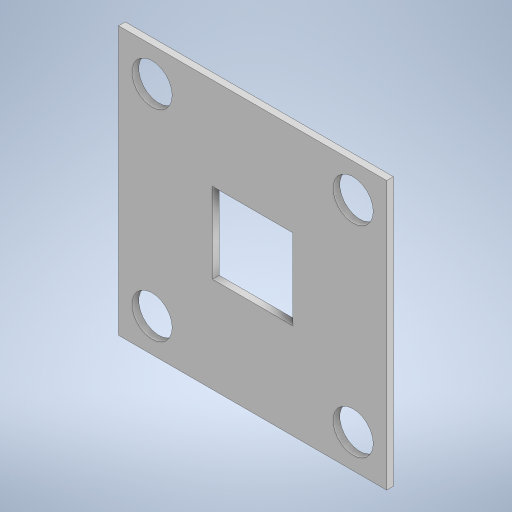
# Autodesk Inventor part: aperture12mm
Saved by Autodesk Inventor 2023 (Build 270158000, 158)
## iProperties
Created: 2022-06-22
Part Number: aperture12mm
Material: Generisch
Document SubType Name: Modeling
Designer: Tim Stechel
Density: 1 g/cm^3
Appearance: Vorgabe
Author: Tim Stechel
Autodesk Inventor part; units mm, degrees
ref_plane "YZ Plane" through (0, 0, 0) normal (1, 0, 0) x (0, 1, 0)
ref_plane "XZ Plane" through (0, 0, 0) normal (0, 1, 0) x (-1, 0, 0)
ref_plane "XY Plane" through (0, 0, 0) normal (0, 0, 1) x (1, 0, 0)
sketch "Skizze1" plane through (0, 0, 0) normal (0, 0, 1) x (1, 0, 0)
  line L0 (0, 0) -> (40, 0)
  line L1 (40, 0) -> (40, 40)
  line L2 (40, 40) -> (0, 40)
  line L3 (0, 40) -> (0, 0)
  circle A0 centre (20, 20.2527) radius 0.3489
  line L4 (0, 40) -> (5, 40)
  line L5 (0, 38.1665) -> (0, 40)
  line L6 (0, 40) -> (5, 40)
  line L7 (5, 40) -> (5, 35)
  line L8 (5, 35) -> (0, 35)
  line L9 (0, 35) -> (0, 40)
  circle A1 centre (5, 35) radius 3
  line L10 (40, 40) -> (35, 40)
  line L11 (35, 40) -> (35, 35)
  line L12 (35, 35) -> (40, 35)
  line L13 (40, 35) -> (40, 40)
  line L14 (0, 0) -> (5, 0)
  line L15 (5, 0) -> (5, 5)
  line L16 (5, 5) -> (0, 5)
  line L17 (0, 5) -> (0, 0)
  line L18 (40, 0) -> (35, 0)
  line L19 (35, 0) -> (35, 5)
  line L20 (35, 5) -> (40, 5)
  line L21 (40, 5) -> (40, 0)
  circle A2 centre (5, 5) radius 3
  circle A3 centre (35, 5) radius 3
  circle A4 centre (35, 35) radius 3
  line L22 (20, 20.2527) -> (20, 26.2527)
  line L23 (20, 26.2527) -> (26, 26.2527)
  line L24 (26, 26.2527) -> (14, 26.2527)
  line L25 (14, 26.2527) -> (14, 14.2527)
  line L26 (14, 14.2527) -> (26, 14.2527)
  line L27 (26, 14.2527) -> (26, 26.2527)
  line L28 (14, 20.2527) -> (26, 20.2527)
  dimension "d0" = 40
  dimension "d1" = 40
  dimension "d4" = 5
  dimension "d5" = 5
  dimension "d6" = 6
  dimension "d7" = 5
  dimension "d8" = 5
  dimension "d9" = 6
  dimension "d10" = 6
  dimension "d11" = 6
  dimension "d12" = 6
  dimension "d13" = 6
  dimension "d14" = 12
  dimension "d15" = 12
  constraints: 58 end point, 12 parallel, 7 horizontal, 7 perpendicular, 5 centre point, 4 coincident, 2 midpoint, 1 vertical, 1 other
  measures "d0" distance of L2.end L1.end
  measures "d1" distance of L0.end L1.end
  measures "d4" distance of L7.end L8.end
  measures "d5" distance of L6.end L7.end
  measures "d6" diameter of A1
  measures "d7" distance of L12.end L11.end
  measures "d8" distance of L14.end L15.end
  measures "d9" diameter of A2
  measures "d10" diameter of A3
  measures "d11" diameter of A4
  measures "d12" distance of L22.start L22.end
  measures "d13" distance of L22.end L23.end
  measures "d14" distance of L26.end L25.end
  measures "d15" distance of L24.end L25.end
extrude "Extrusion1" add sketch "Skizze1" along normal blind 1 contours L3 L16 A2 L15 L0 | L15 A2 L16 L3 L8 A1 L7 L2 L11 A4 L12 L1 L20 A3 L19 L0 | L19 A3 L20 L1 L0 | L3 L2 L7 A1 L8 | L12 A4 L11 L2 L1
